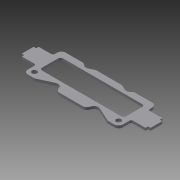
# Autodesk Inventor part: 27030914FacePlate
Saved by Autodesk Inventor 2015 (Build 190159000, 159)
## iProperties
Created: 2014-09-04
Part Number: 27030914FacePlate
Material: Generic
Document SubType Name: Modeling
Designer: STACKPOLE
Density: 1 g/cm^3
Appearance: Default
Author: STACKPOLE
Autodesk Inventor part; units mm, degrees
ref_plane "YZ Plane" through (0, 0, 0) normal (1, 0, 0) x (0, 1, 0)
ref_plane "XZ Plane" through (0, 0, 0) normal (0, 1, 0) x (-1, 0, 0)
ref_plane "XY Plane" through (0, 0, 0) normal (0, 0, 1) x (1, 0, 0)
sketch "Sketch1" plane through (0, 0, 0) normal (0, 0, 1) x (1, 0, 0)
  line L0 (20, 0) -> (133, 0)
  line L1 (153, 8) -> (153, 22)
  line L2 (133, 30) -> (20, 30)
  line L3 (0, 22) -> (0, 8)
  line L4 (150, 25) -> (135, 25)
  line L5 (133, 27) -> (133, 30)
  line L6 (3, 25) -> (18, 25)
  line L7 (20, 27) -> (20, 30)
  line L8 (3, 5) -> (18, 5)
  line L9 (20, 3) -> (20, 0)
  arc A0 (18, 25) -> (20, 27) centre (18, 27) ccw
  arc A1 (20, 3) -> (18, 5) centre (18, 3) ccw
  arc A2 (133, 27) -> (135, 25) centre (135, 27) ccw
  line L10 (150, 5) -> (135, 5)
  line L11 (0, 22) -> (3, 22)
  line L12 (3, 22) -> (3, 25)
  line L13 (0, 8) -> (3, 8)
  line L14 (3, 8) -> (3, 5)
  line L15 (150, 25) -> (150, 22)
  line L16 (150, 22) -> (153, 22)
  line L17 (150, 5) -> (150, 8)
  line L18 (150, 8) -> (153, 8)
  line L19 (133, 0) -> (133, 3)
  arc A3 (135, 5) -> (133, 3) centre (135, 3) ccw
  point P0 (0, 0)
  point P1 (133, 25)
  point P2 (20, 25)
  point P3 (20, 5)
  point P4 (133, 5)
  dimension "d31" = 5
  dimension "d33" = 5
  dimension "d36" = 5
  dimension "d37" = 113
  dimension "d39" = 2
  dimension "d46" = 2
  dimension "d59" = 3
  dimension "d60" = 3
  dimension "d61" = 3
  dimension "d62" = 3
  dimension "d64" = 14
  dimension "d65" = 20
  dimension "d66" = 3
  dimension "d67" = 3
  dimension "d68" = 14
  dimension "d70" = 3
  dimension "d75" = 2
  dimension "d76" = 20
  dimension "d88" = 20
  dimension "d89" = 20
  constraints: 40 end point, 12 point on line, 8 perpendicular, 8 point on circle, 8 tangent, 7 horizontal, 4 centre point, 2 parallel, 2 vertical
  measures "d31" distance of L2.start point (133, 25)
  measures "d33" distance of L2.end point (20, 25)
  measures "d36" distance of L0.start point (20, 5)
  measures "d37" distance of L2.start L2.end
  measures "d39" radius of A0
  measures "d46" radius of A2
  measures "d59" distance of L6.start L11.end
  measures "d60" distance of L3.start L11.end
  measures "d61" distance of L3.end L13.end
  measures "d62" distance of L8.start L13.end
  measures "d64" distance of L3.start L3.end
  measures "d65" distance between parallel lines of L9 L3
  measures "d66" distance of L4.start L15.end
  measures "d67" distance of L15.end L1.end
  measures "d68" distance of L1.start L1.end
  measures "d70" distance of L10.start L17.end
  measures "d75" radius of A3
  measures "d76" distance between parallel lines of L1 L19
  measures "d88" distance between parallel lines of L5 L1
  measures "d89" distance between parallel lines of L3 L7
extrude "Extrusion1" add sketch "Sketch1" along normal blind 3
sketch "Sketch3" plane through (0, 0, 3) normal (0, 0, 1) x (1, 0, 0)
  circle A0 centre (76.5, 15) radius 9
  line L0 (20, 30) -> (133, 30) projected
  line L1 (153, 8) -> (153, 22) projected
  point P0 (0, 0)
  point P1 (2, 30)
  point P2 (151, 30)
  point P3 (153, 2)
  point P4 (153, 28)
  point P5 (27, 30)
  point P6 (126, 30)
  point P7 (153, 7)
  point P8 (153, 23)
  dimension "d24" = 18
  dimension "d25" = 15
  dimension "d26" = 76.5
  constraints: 1 centre point
  measures "d24" diameter of A0
  measures "d25" distance from line of L0 A0.centre
  measures "d26" distance from line of L1 A0.centre
extrude "Extrusion3" cut sketch "Sketch3" against normal through all
sketch "Sketch4" plane through (0, 0, 3) normal (0, 0, 1) x (1, 0, 0)
  circle A0 centre (26.5, -3.5) radius 3
  circle A1 centre (76.5, 15) radius 9 projected
  line L0 (20, 0) -> (55, 0)
  line L1 (33, -10) -> (20, -10)
  line L2 (20, -10) -> (20, 0)
  line L3 (76.5, 0) -> (76.5, 30) construction
  line L4 (133, 30) -> (20, 30) construction
  circle A2 centre (126.5, -3.5) radius 3
  line L5 (133, 0) -> (98, 0)
  line L6 (120, -10) -> (133, -10)
  line L7 (133, -10) -> (133, 0)
  line L8 (33, -10) -> (55, 0)
  line L9 (120, -10) -> (98, 0)
  line L10 (55, 0) -> (59.5455, -10)
  line L11 (98, 0) -> (93.4545, -10)
  line L12 (93.4545, -10) -> (59.5455, -10)
  line L13 (55, 0) -> (98, 0)
  line L14 (133, 0) -> (20, 0) projected
  point P0 (0, 0)
  point P1 (126, 30)
  point P2 (27, 30)
  dimension "d40" = 6
  dimension "d41" = 50
  dimension "d48" = 10
  dimension "d49" = 13
  dimension "d50" = 3.5
  dimension "d54" = 35
  dimension "d55" = 35
  constraints: 26 end point, 4 symmetric about line, 2 centre point, 2 horizontal, 1 collinear, 1 midpoint, 1 parallel, 1 perpendicular, 1 other
  measures "d40" diameter of A0
  measures "d41" horizontal distance of A1.centre A0.centre
  measures "d48" distance of L1.end L0.start
  measures "d49" distance of L1.start L1.end
  measures "d50" distance from line of L0 A0.centre
  measures "d54" distance from line of L0.end L2
  measures "d55" distance from line of L5.end L7
extrude "Extrusion6" add sketch "Sketch4" against normal blind 3 contours L5 L7 L6 L9 | L13 L11 L12 L10 | L0 L8 L1 L2
sketch "Sketch7" plane through (0, 0, 3) normal (0, 0, 1) x (1, 0, 0)
  line L0 (20, 30) -> (20, 35)
  line L1 (20, 35) -> (47.7273, 35)
  line L2 (47.7273, 35) -> (50, 30)
  line L3 (20, 30) -> (133, 30) projected
  line L4 (50, 30) -> (61, 35)
  line L5 (55, 0) -> (59.5455, -10) projected
  line L6 (33, -10) -> (55, 0) projected
  line L7 (133, 30) -> (133, 35)
  line L8 (133, 35) -> (105.2727, 35)
  line L9 (105.2727, 35) -> (103, 30)
  line L10 (103, 30) -> (92, 35)
  line L11 (92, 35) -> (61, 35)
  line L12 (98, 0) -> (120, -10) projected
  line L13 (93.4545, -10) -> (98, 0) projected
  point P0 (0, 0)
  point P1 (57.069, -4.5518)
  point P2 (58.2132, -7.069)
  point P3 (33.986, -9.5518)
  point P4 (50.4482, -2.069)
  point P5 (102.5518, -2.069)
  point P6 (119.014, -9.5518)
  point P7 (94.7868, -7.069)
  point P8 (95.931, -4.5518)
  dimension "d80" = 5
  dimension "d81" = 30
  dimension "d82" = 30
  constraints: 18 end point, 4 parallel, 4 point on line, 2 perpendicular, 2 vertical, 1 collinear, 1 horizontal
  measures "d80" distance of L0.start L0.end
  measures "d81" distance of L0.start L2.end
  measures "d82" distance from line of L7 L9.end
extrude "Extrusion7" add sketch "Sketch7" against normal blind 3
fillet "Fillet4" radius 5 2 edges at (50, 30, 1.5) (103, 30, 1.5)
fillet "Fillet5" radius 5 2 edges at (55, 0, 1.5) (98, 0, 1.5)
fillet "Fillet6" radius 5 12 edges at (20, -10, 1.5) (20, 35, 1.5) (47.7273, 35, 1.5) (61, 35, 1.5) (92, 35, 1.5) (105.2727, 35, 1.5) (133, 35, 1.5) (133, -10, 1.5) (120, -10, 1.5) (93.4545, -10, 1.5) (59.5455, -10, 1.5) (33, -10, 1.5)
sketch "Sketch10" plane through (0, 0, 0) normal (0, 0, -1) x (-1, 0, 0)
  line L0 (-123.5, 2.5) -> (-29.5, 2.5)
  line L1 (-26.5, 5.5) -> (-26.5, 24.5)
  line L2 (-29.5, 27.5) -> (-123.5, 27.5)
  line L3 (-126.5, 24.5) -> (-126.5, 5.5)
  circle A0 centre (-76.5, 15) radius 9 projected
  line L4 (-126.5, 2.5) -> (-26.5, 27.5) construction
  line L5 (-26.5, 2.5) -> (-126.5, 27.5) construction
  arc A1 (-123.5, 27.5) -> (-126.5, 24.5) centre (-123.5, 24.5) ccw
  arc A2 (-26.5, 24.5) -> (-29.5, 27.5) centre (-29.5, 24.5) ccw
  arc A3 (-29.5, 2.5) -> (-26.5, 5.5) centre (-29.5, 5.5) ccw
  arc A4 (-126.5, 5.5) -> (-123.5, 2.5) centre (-123.5, 5.5) ccw
  point P0 (0, 0)
  dimension "d90" = 25
  dimension "d91" = 100
  dimension "d92" = 3
  constraints: 12 end point, 8 point on circle, 8 point on line, 8 tangent, 4 centre point, 3 equal radius, 2 midpoint, 2 parallel, 1 horizontal, 1 perpendicular
  measures "d90" distance of L5.end L4.start
  measures "d91" distance of L4.end L5.end
  measures "d92" radius of A1
extrude "Extrusion8" cut sketch "Sketch10" against normal through all
body "Solid1"
